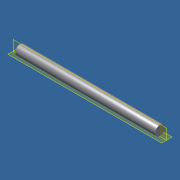
# Autodesk Inventor part: Update_SetBaseQuantity
Saved by Autodesk Inventor 2012 SP1 (Build 160190100, 190)
## iProperties
Created: 2011-11-09
Part Number: Update_SetBaseQuantity
Material: P792.4
Document SubType Name: Modeling
Designer: bleasure
Density: 8.08 g/cm^3
RuleStatus: InUse
AfterMaterialChange0: file://BarMaterial
AfterMaterialChange1: file://CoilMaterial
AfterMaterialChange2: file://GlassRailMaterial
AfterMaterialChange3: file://PipeMaterial
AfterMaterialChange4: file://SheetMaterial
AfterMaterialChange5: file://TubeMaterial
Finish: #4 Satin
MaterialDescription: 1-1/4 Schd 40 Pipe 304 SS 1.66 OD .140 Wall 21 Ft.
igesFile: none.igs
Length: 0
Author: bleasure
Revision Number: 1
Autodesk Inventor part; units mm, degrees
ref_plane "YZ Plane" through (0, 0, 0) normal (1, 0, 0) x (0, 1, 0)
sketch "1.90 Caprail" plane through (0, 0, 0) normal (0, 0, 1) x (1, 0, 0)
  line L0 (-57.7384, 25.6152) -> (-57.7384, 36.7912) construction
  arc A0 (-65.9934, 36.7912) -> (-67.5174, 35.2672) centre (-65.9934, 35.2672) ccw
  arc A1 (-47.9594, 35.2672) -> (-49.4834, 36.7912) centre (-49.4834, 35.2672) ccw
  arc A2 (-69.8345, 6.4876) -> (-69.016, 6.9384) centre (-69.5494, 6.9384) ccw
  line L1 (-69.016, 6.9384) -> (-69.016, 35.2672)
  arc A3 (-65.9934, 38.2898) -> (-69.016, 35.2672) centre (-65.9934, 35.2672) ccw
  line L2 (-65.9934, 38.2898) -> (-49.4834, 38.2898)
  arc A4 (-46.4608, 35.2672) -> (-49.4834, 38.2898) centre (-49.4834, 35.2672) ccw
  line L3 (-46.4608, 35.2672) -> (-46.4608, 6.9384)
  arc A5 (-46.4608, 6.9384) -> (-45.6423, 6.4876) centre (-45.9274, 6.9384) ccw
  arc A6 (-45.6423, 6.4876) -> (-69.8345, 6.4876) centre (-57.7384, 25.6152) ccw
  line L4 (-47.9594, 6.9384) -> (-47.9594, 35.2672)
  line L5 (-49.4834, 36.7912) -> (-65.9934, 36.7912)
  line L6 (-67.5174, 35.2672) -> (-67.5174, 6.9384)
  arc A7 (-70.5058, 5.1455) -> (-67.5174, 6.9384) centre (-69.5494, 6.9384) ccw
  arc A8 (-47.9594, 6.9384) -> (-44.9711, 5.1455) centre (-45.9274, 6.9384) ccw
  arc A9 (-70.5083, 5.1411) -> (-44.9685, 5.1411) centre (-57.7384, 25.6152) ccw
  circle A10 centre (-57.7384, 25.6152) radius 24.13 construction
  arc A11 (-70.5058, 5.1455) -> (-70.5083, 5.1411) centre (-70.507, 5.1433) ccw
  arc A12 (-44.9685, 5.1411) -> (-44.9711, 5.1455) centre (-44.9699, 5.1433) ccw
  point P0 (-47.9594, 36.7912)
  point P1 (-67.5174, 36.7912)
  dimension "d0" = 48.26
  dimension "d1" = 19.558
  dimension "d2" = 2.032
  dimension "d3" = 11.176
  dimension "d4" = 1.524
  dimension "d5" = 1.4986
  dimension "d6" = 0.0025
  measures "d0" diameter of A10
  measures "d1" distance of point (-47.959, 36.791) point (-67.517, 36.791)
  measures "d2" radius of A8
  measures "d3" distance of L0.start L0.end
  measures "d4" radius of A0
  measures "d5" distance between parallel lines of L3 L4
  measures "d6" radius of A11
sketch "1.66 Caprail" plane through (0, 0, 0) normal (0, 0, 1) x (1, 0, 0)
  arc A0 (55.7245, -3.4499) -> (81.6283, -3.4499) centre (68.6764, 13.1843) ccw
  arc A1 (55.7275, -3.4458) -> (58.8974, -1.7623) centre (56.8654, -1.7623) ccw
  arc A2 (78.4554, -1.7623) -> (81.6253, -3.4458) centre (80.4874, -1.7623) ccw
  line L0 (58.8974, -1.7623) -> (58.8974, 20.8043)
  line L1 (60.4214, 22.3283) -> (76.9314, 22.3283)
  line L2 (78.4554, 20.8043) -> (78.4554, -1.7623)
  line L3 (68.6764, 22.3283) -> (68.6764, 13.1843) construction
  arc A3 (60.4214, 22.3283) -> (58.8974, 20.8043) centre (60.4214, 20.8043) ccw
  arc A4 (78.4554, 20.8043) -> (76.9314, 22.3283) centre (76.9314, 20.8043) ccw
  arc A5 (79.954, -1.7623) -> (80.8181, -2.1808) centre (80.4874, -1.7623) ccw
  line L4 (79.954, -1.7623) -> (79.954, 20.8043)
  arc A6 (79.954, 20.8043) -> (76.9314, 23.8269) centre (76.9314, 20.8043) ccw
  line L5 (76.9314, 23.8269) -> (60.4214, 23.8269)
  arc A7 (60.4214, 23.8269) -> (57.3988, 20.8043) centre (60.4214, 20.8043) ccw
  line L6 (57.3988, 20.8043) -> (57.3988, -1.7623)
  arc A8 (56.5347, -2.1808) -> (57.3988, -1.7623) centre (56.8654, -1.7623) ccw
  arc A9 (80.8181, -2.1808) -> (56.5347, -2.1808) centre (68.6764, 13.1843) ccw
  circle A10 centre (68.6764, 13.1843) radius 21.082 construction
  arc A11 (55.7275, -3.4458) -> (55.7245, -3.4499) centre (55.7261, -3.4479) ccw
  arc A12 (81.6283, -3.4499) -> (81.6253, -3.4458) centre (81.6268, -3.4479) ccw
  point P0 (58.8974, 22.3283)
  point P1 (78.4554, 22.3283)
  dimension "d7" = 42.164
  dimension "d8" = 19.558
  dimension "d9" = 9.144
  dimension "d10" = 2.032
  dimension "d11" = 1.524
  dimension "d12" = 1.4986
  dimension "d13" = 0.0025
  measures "d7" diameter of A10
  measures "d8" distance of point (58.897, 22.328) point (78.455, 22.328)
  measures "d9" distance of L3.start L3.end
  measures "d10" radius of A1
  measures "d11" radius of A3
  measures "d12" distance between parallel lines of L2 L4
  measures "d13" radius of A11
sketch "1.50 Caprail" plane through (0, 0, 0) normal (0, 0, 1) x (1, 0, 0)
  arc A0 (154.6368, -0.6357) -> (180.8596, -0.6357) centre (167.7482, 13.1843) ccw
  arc A1 (154.6402, -0.6319) -> (157.9692, 0.9323) centre (155.9372, 0.9323) ccw
  arc A2 (177.5272, 0.9323) -> (180.8562, -0.6319) centre (179.5592, 0.9323) ccw
  circle A3 centre (167.7482, 13.1843) radius 19.05 construction
  arc A4 (179.0258, 0.9323) -> (179.9294, 0.5483) centre (179.5592, 0.9323) ccw
  line L0 (179.0258, 0.9323) -> (179.0258, 23.0903)
  arc A5 (179.0258, 23.0903) -> (176.0032, 26.1129) centre (176.0032, 23.0903) ccw
  line L1 (176.0032, 26.1129) -> (159.4932, 26.1129)
  arc A6 (159.4932, 26.1129) -> (156.4706, 23.0903) centre (159.4932, 23.0903) ccw
  line L2 (156.4706, 23.0903) -> (156.4706, 0.9323)
  arc A7 (155.567, 0.5483) -> (156.4706, 0.9323) centre (155.9372, 0.9323) ccw
  arc A8 (179.9294, 0.5483) -> (155.567, 0.5483) centre (167.7482, 13.1843) ccw
  line L3 (157.9692, 0.9323) -> (157.9692, 23.0903)
  line L4 (159.4932, 24.6143) -> (176.0032, 24.6143)
  line L5 (177.5272, 23.0903) -> (177.5272, 0.9323)
  arc A9 (159.4932, 24.6143) -> (157.9692, 23.0903) centre (159.4932, 23.0903) ccw
  arc A10 (177.5272, 23.0903) -> (176.0032, 24.6143) centre (176.0032, 23.0903) ccw
  line L6 (167.7482, 24.6143) -> (167.7482, 13.1843) construction
  arc A11 (154.6402, -0.6319) -> (154.6368, -0.6357) centre (154.6385, -0.6339) ccw
  arc A12 (180.8596, -0.6357) -> (180.8562, -0.6319) centre (180.8578, -0.6339) ccw
  point P0 (157.9692, 24.6143)
  point P1 (177.5272, 24.6143)
  dimension "d14" = 38.1
  dimension "d15" = 19.558
  dimension "d16" = 2.032
  dimension "d17" = 1.524
  dimension "d18" = 11.43
  dimension "d19" = 1.4986
  dimension "d20" = 0.0025
  measures "d14" diameter of A3
  measures "d15" distance of point (157.969, 24.614) point (177.527, 24.614)
  measures "d16" radius of A1
  measures "d17" radius of A9
  measures "d18" distance of L6.start L6.end
  measures "d19" distance between parallel lines of L2 L3
  measures "d20" radius of A11
sketch "1.90 Caprail Outside Edge" plane through (0, 0, 0) normal (0, 0, 1) x (1, 0, 0)
  arc A0 (8.6191, 38.6174) -> (-17.175, 38.6174) centre (-4.278, 59.0116) ccw
  line L0 (5.501, 40.3348) -> (5.501, 68.5975)
  line L1 (3.977, 70.1215) -> (-12.533, 70.1215)
  line L2 (-14.057, 68.5975) -> (-14.057, 40.3348)
  line L3 (-4.278, 59.0116) -> (-4.278, 70.1215) construction
  arc A1 (-17.175, 38.6174) -> (-14.057, 40.3348) centre (-16.089, 40.3348) ccw
  arc A2 (5.501, 40.3348) -> (8.6191, 38.6174) centre (7.533, 40.3348) ccw
  arc A3 (-12.533, 70.1215) -> (-14.057, 68.5975) centre (-12.533, 68.5975) ccw
  arc A4 (5.501, 68.5975) -> (3.977, 70.1215) centre (3.977, 68.5975) ccw
  point P0 (5.501, 70.1215)
  point P1 (-14.057, 70.1215)
  point P2 (-14.057, 36.9519)
  point P3 (5.501, 36.9519)
  dimension "d21" = 13.02
  dimension "d22" = 19.558
  dimension "d23" = 24.13
  dimension "d24" = 2.032
  dimension "d25" = 1.524
  measures "d21" distance edge to line of A0 L1
  measures "d22" distance of point (5.501, 70.122) point (-14.057, 70.122)
  measures "d23" radius of A0
  measures "d24" radius of A1
  measures "d25" radius of A3
sketch "1.66 Caprail Outside Edge" plane through (0, 0, 0) normal (0, 0, 1) x (1, 0, 0)
  arc A0 (-64.2087, 6.8983) -> (-90.3503, 6.8983) centre (-77.2795, 23.4393) ccw
  line L0 (-67.5005, 8.4926) -> (-67.5005, 30.9932)
  line L1 (-69.0245, 32.5172) -> (-85.5345, 32.5172)
  line L2 (-87.0585, 30.9932) -> (-87.0585, 8.4926)
  line L3 (-77.2795, 23.4393) -> (-77.2795, 32.5172) construction
  arc A1 (-90.3503, 6.8983) -> (-87.0585, 8.4926) centre (-89.0905, 8.4926) ccw
  arc A2 (-67.5005, 8.4926) -> (-64.2087, 6.8983) centre (-65.4685, 8.4926) ccw
  arc A3 (-85.5345, 32.5172) -> (-87.0585, 30.9932) centre (-85.5345, 30.9932) ccw
  arc A4 (-67.5005, 30.9932) -> (-69.0245, 32.5172) centre (-69.0245, 30.9932) ccw
  point P0 (-67.5005, 32.5172)
  point P1 (-87.0585, 32.5172)
  point P2 (-87.0585, 4.7625)
  point P3 (-67.5005, 4.7625)
  dimension "d26" = 12.004
  dimension "d27" = 19.558
  dimension "d28" = 21.082
  dimension "d29" = 2.032
  dimension "d30" = 1.524
  measures "d26" distance edge to line of A0 L1
  measures "d27" distance of point (-67.501, 32.517) point (-87.059, 32.517)
  measures "d28" radius of A0
  measures "d29" radius of A1
  measures "d30" radius of A3
sketch "1.50 Caprail Outside Edge" plane through (0, 0, 0) normal (0, 0, 1) x (1, 0, 0)
  arc A0 (-129.2922, 11.7711) -> (-155.7348, 11.7711) centre (-142.5135, 25.486) ccw
  line L0 (-132.7345, 13.234) -> (-132.7345, 35.4784)
  line L1 (-134.2585, 37.0024) -> (-150.7685, 37.0024)
  line L2 (-152.2925, 35.4784) -> (-152.2925, 13.234)
  line L3 (-142.5135, 25.486) -> (-142.5135, 37.0024) construction
  arc A1 (-155.7348, 11.7711) -> (-152.2925, 13.234) centre (-154.3245, 13.234) ccw
  arc A2 (-132.7345, 13.234) -> (-129.2922, 11.7711) centre (-130.7025, 13.234) ccw
  arc A3 (-150.7685, 37.0024) -> (-152.2925, 35.4784) centre (-150.7685, 35.4784) ccw
  arc A4 (-132.7345, 35.4784) -> (-134.2585, 37.0024) centre (-134.2585, 35.4784) ccw
  point P0 (-132.7345, 37.0024)
  point P1 (-152.2925, 37.0024)
  point P2 (-152.2925, 9.1375)
  point P3 (-132.7345, 9.1375)
  dimension "d31" = 7.5336
  dimension "d32" = 19.558
  dimension "d33" = 19.05
  dimension "d34" = 2.032
  dimension "d35" = 1.524
  measures "d31" distance edge to line of A0 L1
  measures "d32" distance of point (-132.734, 37.002) point (-152.292, 37.002)
  measures "d33" radius of A0
  measures "d34" radius of A1
  measures "d35" radius of A3
sketch "Sketch1" plane through (0, 0, 0) normal (0, 0, 1) x (1, 0, 0)
  line L0 (0, 0) -> (609.6, 0)
  line L1 (609.6, 0) -> (609.6, 42.164)
  line L2 (609.6, 42.164) -> (0, 42.164)
  line L3 (0, 42.164) -> (0, 0)
  dimension "d37" = 42.164
  dimension "d38" = 609.6
  constraints: 8 end point, 2 parallel, 1 horizontal, 1 perpendicular
  measures "d37" distance between parallel lines of L0 L2
  measures "d38" distance of L1.end L2.end
extrude "Extrusion1" add sketch "Sketch1" along normal mid plane 42.164
fillet "Fillet1" radius 21.082 4 edges at (304.8, 42.164, -21.082) (304.8, 42.164, 21.082) (304.8, 0, -21.082) (304.8, 0, 21.082)
equation "\"d37\" = PipeOD"
equation "\"d39\" = PipeOD"
equation "\"d41\" = 0.5 * PipeOD"
equation "\"PipeOD\" = 42.164"
equation "\"PipeWallThickness\" = 3.556"
equation "\"Length\" = 609.6"
body "Solid1"
